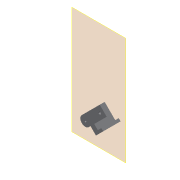
# Autodesk Inventor part: 30_CUBE_openSIM_Laserarm
Saved by Autodesk Inventor 2019 (Build 230136000, 136)
## iProperties
Created: 2019-08-01
Part Number: 30_CUBE_openSIM_Laserarm
Material: Generic
Document SubType Name: Modeling
Designer: diederichbenedict
Density: 1 g/cm^3
Appearance: Default
Author: diederichbenedict
Autodesk Inventor part; units mm, degrees
ref_plane "YZ Plane" through (0, 0, 0) normal (1, 0, 0) x (0, 1, 0)
ref_plane "XZ Plane" through (0, 0, 0) normal (0, 1, 0) x (-1, 0, 0)
ref_plane "XY Plane" through (0, 0, 0) normal (0, 0, 1) x (1, 0, 0)
ref_plane "Work Plane1" through (0, 0, 0) normal (0, 0, 1) x (1, 0, 0)
sketch "Sketch1" plane through (0, 0, 0) normal (0, 0, 1) x (1, 0, 0)
  line L0 (-41.9, 57.6) -> (-41.9, 91.9) construction
  line L1 (-41.9, -91.9) -> (41.9, -91.9) construction
  line L2 (-7.4, -59.4) -> (-7.4, -67.3) construction
  circle A0 centre (-24.65, -74.65) radius 17.25 construction
  circle A1 centre (-24.65, -74.65) radius 6.3062 construction
  circle A2 centre (-24.65, -74.65) radius 1.9
  line L3 (-24.65, -74.65) -> (11.6672, -38.3328) construction
  line L4 (-17.5789, -81.7211) -> (18.7383, -45.4039)
  line L5 (4.5961, -31.2617) -> (-31.7211, -67.5789)
  arc A3 (-31.7211, -67.5789) -> (-17.5789, -81.7211) centre (-24.65, -74.65) ccw
  arc A4 (18.7383, -45.4039) -> (4.5961, -31.2617) centre (11.6672, -38.3328) ccw construction
  circle A5 centre (11.6672, -38.3328) radius 2.6562
  line L6 (4.5961, -31.2617) -> (12.137, -23.7208)
  line L7 (3.5996, -14.8432) -> (9.3348, -8.7305) construction
  line L8 (33.237, -42.6502) -> (38.9722, -36.5375) construction
  line L9 (12.137, -23.7208) -> (33.5765, -45.1603) construction
  line L10 (33.5765, -45.1603) -> (12.137, -23.7208)
  line L11 (18.7383, -45.4039) -> (29.8258, -56.4914)
  line L12 (29.8258, -56.4914) -> (44.5482, -41.7691)
  line L13 (44.5482, -41.7691) -> (40.758, -37.9789)
  line L14 (40.758, -37.9789) -> (33.5765, -45.1603)
  point P0 (0, 0)
  point P1 (41.9, -91.9)
  point P2 (-6.4914, -56.4914)
  dimension "d0" = 3.8
  dimension "d3" = 10
  dimension "d4" = 45
  dimension "d5" = 40.64
  dimension "d6" = 20.32
  constraints: 22 end point, 7 tangent, 6 centre point, 4 point on circle, 3 coincident, 3 perpendicular, 2 parallel, 1 collinear, 1 midpoint
  measures "d0" diameter of A2
  measures "d3" radius of A3
  measures "d4" angle of L0 L3
  measures "d5" distance between parallel lines of L8 L7
  measures "d6" distance from line of L14 L3.end
extrude "Extrusion1" add sketch "Sketch1" along normal blind 10
sketch "Sketch2" plane through (0, 0, 10) normal (0, 0, 1) x (1, 0, 0)
  circle A0 centre (-24.65, -74.65) radius 1.9 projected
  circle A1 centre (11.6672, -38.3328) radius 2.6562 projected
  line L0 (-17.5789, -81.7211) -> (18.7383, -45.4039) projected
  line L1 (18.7383, -45.4039) -> (29.8258, -56.4914) projected
  line L2 (29.8258, -56.4914) -> (44.5482, -41.7691) projected
  line L3 (44.5482, -41.7691) -> (40.758, -37.9789) projected
  line L4 (40.758, -37.9789) -> (33.5765, -45.1603) projected
  line L5 (33.5765, -45.1603) -> (12.137, -23.7208) projected
  line L6 (12.137, -23.7208) -> (-31.7211, -67.5789) projected
  arc A2 (-31.7211, -67.5789) -> (-17.5789, -81.7211) centre (-24.65, -74.65) ccw projected
  line L7 (44.5482, -41.7691) -> (40.758, -37.9789) projected
  line L8 (44.5482, -41.7691) -> (40.758, -37.9789)
  line L9 (40.758, -37.9789) -> (26.0356, -52.7012)
  line L10 (26.0356, -52.7012) -> (29.8258, -56.4914)
  line L11 (29.8258, -56.4914) -> (44.5482, -41.7691)
  line L12 (18.7383, -45.4039) -> (29.8258, -56.4914) projected
  line L13 (26.0356, -52.7012) -> (18.7383, -45.4039)
  line L14 (18.7383, -45.4039) -> (26.2792, -37.863)
  line L15 (26.2792, -37.863) -> (33.5765, -45.1603)
  line L16 (33.5765, -45.1603) -> (26.0356, -52.7012)
  point P0 (0, 0)
  constraints: 16 end point, 5 equal length, 3 perpendicular
extrude "Extrusion2" add sketch "Sketch2" along normal blind 25.4 contours L14 L5 L9 L1 | L9 L4 L3 L2 L1
sketch "Sketch3" plane through (44.5482, -41.7691, 35.4) normal (0.7071068, -0.7071068, 0) x (-0.7071068, -0.7071068, 0)
  circle A0 centre (5.6027, 15.08) radius 1.25
  line L0 (20.8205, 35.4) -> (0, 35.4) projected
  point P0 (1.9651, 35.4)
  dimension "d9" = 2.5
  dimension "d10" = 20.32
  constraints: 1 centre point
  measures "d9" diameter of A0
  measures "d10" distance from line of A0.centre L0
extrude "Extrusion3" cut sketch "Sketch3" against normal blind 25.4
sketch "Sketch4" plane through (-17.5789, -81.7211, 10) normal (0.7071068, -0.7071068, 0) x (-0.7071068, -0.7071068, 0)
  line L0 (10, 10) -> (10, 0) projected
  line L1 (10, 7.3414) -> (-12.1363, 7.3414)
  line L2 (-14.7676, 5.9432) -> (-18.7808, 0)
  line L3 (0, 0) -> (-51.3603, 0) projected
  arc A0 (-12.1363, 7.3414) -> (-14.7676, 5.9432) centre (-12.1363, 4.1664) ccw
  line L4 (-18.7808, 0) -> (10, 0)
  line L5 (10, 7.3414) -> (10, 0)
  point P0 (-70.2157, 10)
  dimension "d13" = 3.175
  constraints: 8 end point, 2 horizontal, 2 point on circle, 2 point on line, 2 tangent, 1 centre point, 1 collinear
  measures "d13" radius of A0
extrude "Extrusion4" cut sketch "Sketch4" against normal blind 25.4
body "Solid1"
